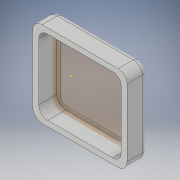
# Autodesk Inventor part: GoPro_Cap_Lens
Saved by Autodesk Inventor 2019 (Build 230136000, 136)
## iProperties
Created: 2019-02-06
Part Number: GoPro_Cap_Lens
Material: Generic
Document SubType Name: Modeling
Designer: jmc
Density: 1 g/cm^3
Appearance: Default
Author: jmc
## iProperties of the stored document GoPro_Cap_Lens_3DPrint.ipt
Created: 2019-02-06
Part Number: GoPro_Cap_Lens_3DPrint
Material: Generic
Document SubType Name: Modeling
Designer: assman
Density: 1 g/cm^3
Appearance: Default
Author: assman
Autodesk Inventor part; units mm, degrees
ref_plane "YZ Plane" through (0, 0, 0) normal (1, 0, 0) x (0, 1, 0)
ref_plane "XZ Plane" through (0, 0, 0) normal (0, 1, 0) x (-1, 0, 0)
ref_plane "XY Plane" through (0, 0, 0) normal (0, 0, 1) x (1, 0, 0)
sketch "Sketch1" plane through (-3.508, -14.003, 0) normal (0, 0, 1) x (1, 0, 0)
  line L0 (-3.495, 25.79953) -> (-3.495, 3.514145)
  line L1 (28.510999, 26.087) -> (28.510999, 3.154266)
  line L2 (0.019145, 0) -> (25.356733, 0)
  line L3 (25.487768, 29.005968) -> (-0.274, 29.005968)
  arc A0 (-3.495, 3.514145) -> (0.019145, 0) centre (0.019145, 3.514145) ccw
  arc A1 (25.356733, 0) -> (28.510999, 3.154266) centre (25.356733, 3.154266) ccw
  arc A2 (28.510999, 25.98277) -> (25.487768, 29.005968) centre (25.487768, 25.982737) ccw
  arc A3 (-0.274, 29.005968) -> (-3.495, 25.79953) centre (-0.288529, 25.79953) ccw
  line L4 (9.854411, 29.005968) -> (9.854411, 34.005968) construction
  point P0 (12.606884, 14.620633)
  dimension "d0" = 5
  constraints: 10 end point, 8 point on circle, 4 centre point, 2 point on line, 2 tangent, 1 vertical
  measures "d0" distance of L4.start L4.end
sketch "Sketch3" plane through (0, 0, 0) normal (0, 0, 1) x (1, 0, 0)
  arc A0 (-5.67549, 17.117612) -> (-9.369977, 13.439828) centre (-5.692155, 13.439828) ccw
  line L0 (-9.369977, 13.439828) -> (-9.369977, -12.121509)
  arc A1 (-9.369977, -12.121509) -> (-5.339252, -16.152233) centre (-5.339252, -12.121509) ccw
  line L1 (-5.339252, -16.152233) -> (23.722961, -16.152233)
  arc A2 (23.722961, -16.152233) -> (27.340904, -12.53429) centre (23.722961, -12.53429) ccw
  line L2 (27.340904, 13.769556) -> (27.340904, -12.53429)
  arc A3 (27.340904, 13.650004) -> (23.873258, 17.117612) centre (23.873258, 13.649966) ccw
  line L3 (23.873258, 17.117612) -> (-5.67549, 17.117612)
  point P0 (0, 0)
  point P1 (25.002999, 11.97977)
  point P2 (9.098884, 0.617633)
  constraints: 8 end point, 8 point on circle, 4 centre point, 1 point on line
extrude "Extrusion1" add sketch "Sketch3" along normal blind 7.886
shell "Shell1" thickness 2.5 removed faces 1 at (4.286172, 6.027663, 7.886)
ref_plane "Work Plane3" through (-5.682724, 14.617612, 2.5) normal (0, 0, 1) x (1, 0, 0)
sketch "Sketch4" plane through (-5.682724, 14.617612, 2.5) normal (0, 0, 1) x (1, 0, 0)
  point P0 (5.682724, -14.617612)
extrude "Extrusion2" cut sketch "Sketch1" along normal blind 21
sketch "Sketch5" plane through (-5.682724, 14.617612, 2.5) normal (0, 0, 1) x (1, 0, 0)
  arc A0 (0.362072, 0) -> (-1.187253, -1.907094) centre (1.886195, -2.821082) ccw
  line L0 (0.362072, 0) -> (0, 0)
  arc A1 (0, 0) -> (-1.187253, -1.177784) centre (-0.009431, -1.177784) ccw
  line L1 (-1.187253, -1.177784) -> (-1.187253, -1.907094)
  arc A2 (-1.187253, -26.064188) -> (0.663427, -28.269845) centre (2.19387, -25.106467) ccw
  line L2 (-1.187253, -26.064188) -> (-1.187253, -26.73912)
  arc A3 (-1.187253, -26.73912) -> (0.343472, -28.269845) centre (0.343472, -26.73912) ccw
  line L3 (0.343472, -28.269845) -> (0.663427, -28.269845)
  arc A4 (28.977067, -28.269845) -> (30.523628, -26.464498) centre (27.531457, -25.466346) ccw
  line L4 (28.977067, -28.269845) -> (29.405685, -28.269845)
  arc A5 (29.405685, -28.269845) -> (30.523628, -27.151902) centre (29.405685, -27.151902) ccw
  line L5 (30.523628, -27.151902) -> (30.523628, -26.464498)
  arc A6 (30.523628, -1.661234) -> (29.139496, 0) centre (27.662493, -2.637875) ccw
  line L6 (30.523628, -1.661234) -> (30.523628, -0.967608)
  arc A7 (30.523628, -0.967608) -> (29.555982, 0) centre (29.555983, -0.967646) ccw
  line L7 (29.555982, 0) -> (29.139496, 0)
  point P0 (5.682724, -14.617612)
extrude "Extrusion3" add sketch "Sketch5" along normal up to surface (5.386 mm away)
sketch "Sketch6" plane through (-5.682724, 14.617612, 2.5) normal (0, 0, 1) x (1, 0, 0)
  arc A0 (27.531457, -28.620612) -> (30.685723, -25.466346) centre (27.531457, -25.466346) ccw
  line L0 (2.19387, -28.620612) -> (27.531457, -28.620612)
  arc A1 (-1.320276, -25.106467) -> (2.19387, -28.620612) centre (2.19387, -25.106467) ccw
  line L1 (-1.320276, -2.821082) -> (-1.320276, -25.106467)
  arc A2 (1.900724, 0.385356) -> (-1.320276, -2.821082) centre (1.886195, -2.821082) ccw
  line L2 (27.662492, 0.385356) -> (1.900724, 0.385356)
  arc A3 (30.685723, -2.637842) -> (27.662492, 0.385356) centre (27.662493, -2.637875) ccw
  line L3 (30.685723, -25.466346) -> (30.685723, -2.637842)
  point P0 (5.682724, -14.617612)
extrude "Extrusion4" add sketch "Sketch6" against normal up to surface (2.5 mm away)
sketch "Sketch7" plane through (-5.682724, 14.617612, 2.5) normal (0, 0, 1) x (1, 0, 0)
  arc A0 (27.531457, -28.620612) -> (30.685723, -25.466346) centre (27.531457, -25.466346) ccw
  line L0 (30.685723, -2.637842) -> (30.685723, -25.466346)
  arc A1 (30.685723, -2.637842) -> (27.662492, 0.385356) centre (27.662493, -2.637875) ccw
  line L1 (1.900724, 0.385356) -> (27.662492, 0.385356)
  arc A2 (1.900724, 0.385356) -> (-1.320276, -2.821082) centre (1.886195, -2.821082) ccw
  line L2 (-1.320276, -25.106467) -> (-1.320276, -2.821082)
  arc A3 (-1.320276, -25.106467) -> (2.19387, -28.620612) centre (2.19387, -25.106467) ccw
  line L3 (27.531457, -28.620612) -> (2.19387, -28.620612)
  arc A4 (1.896794, -1.114644) -> (0.179724, -2.821082) centre (1.886195, -2.821082) ccw
  line L4 (1.896794, -1.114644) -> (27.662493, -1.114644)
  arc A5 (29.185723, -2.637875) -> (27.662493, -1.114644) centre (27.662493, -2.637875) ccw
  line L5 (29.185723, -2.637875) -> (29.185723, -25.466346)
  arc A6 (27.531457, -27.120612) -> (29.185723, -25.466346) centre (27.531457, -25.466346) ccw
  line L6 (27.531457, -27.120612) -> (2.19387, -27.120612)
  arc A7 (0.179724, -25.106467) -> (2.19387, -27.120612) centre (2.19387, -25.106467) ccw
  line L7 (0.179724, -25.106467) -> (0.179724, -2.821082)
  point P0 (5.682724, -14.617612)
  dimension "d11" = 1.5
  constraints: 8 end point, 8 point on circle, 4 centre point, 7 other
  measures "d11" radial gap between concentric circles of A2 A4
extrude "Extrusion5" cut sketch "Sketch7" against normal blind 21 contours L4 A5 L5 A6 L6 A7 L7 A4
sketch "Sketch8" plane through (-5.682724, 14.617612, 2.5) normal (0, 0, 1) x (1, 0, 0)
  line L0 (0.179724, -25.106467) -> (0.179724, -2.821082)
  arc A0 (1.896794, -1.114644) -> (0.179724, -2.821082) centre (1.886195, -2.821082) ccw
  line L1 (1.896794, -1.114644) -> (27.662493, -1.114644)
  arc A1 (29.185723, -2.637875) -> (27.662493, -1.114644) centre (27.662493, -2.637875) ccw
  line L2 (29.185723, -2.637875) -> (29.185723, -25.466346)
  arc A2 (27.531457, -27.120612) -> (29.185723, -25.466346) centre (27.531457, -25.466346) ccw
  line L3 (27.531457, -27.120612) -> (2.19387, -27.120612)
  arc A3 (0.179724, -25.106467) -> (2.19387, -27.120612) centre (2.19387, -25.106467) ccw
  arc A4 (27.531457, -28.620612) -> (30.685723, -25.466346) centre (27.531457, -25.466346) ccw
  line L4 (30.685723, -2.637842) -> (30.685723, -25.466346)
  arc A5 (30.685723, -2.637842) -> (27.662492, 0.385356) centre (27.662493, -2.637875) ccw
  line L5 (1.900724, 0.385356) -> (27.662492, 0.385356)
  arc A6 (1.900724, 0.385356) -> (-1.320276, -2.821082) centre (1.886195, -2.821082) ccw
  line L6 (-1.320276, -25.106467) -> (-1.320276, -2.821082)
  arc A7 (-1.320276, -25.106467) -> (2.19387, -28.620612) centre (2.19387, -25.106467) ccw
  line L7 (27.531457, -28.620612) -> (2.19387, -28.620612)
  point P0 (5.682724, -14.617612)
extrude "Extrusion6" cut sketch "Sketch8" against normal blind 1.6
fillet "Fillet1" radius 2 8 edges at (26.3252, 16.102, 0) (27.3409, 0.5579, 0) (26.2812, -15.0926, 0) (9.1919, -16.1522, 0) (-8.1894, -14.9717, 0) (-9.37, 0.6592, 0) (-8.2869, 16.0463, 0) (9.0989, 17.1176, 0)
fillet "Fillet1" radius 1 8 edges at (9.0969, 13.503, 0) (23.503, 0.5655, 0) (23.0185, -12.0185, 0) (9.1799, -12.503, 0) (-4.9131, -11.9131, 0) (-5.503, 0.6538, 0) (-4.9994, 13.0069, 0) (23.0569, 13.0568, 0)
body "Solid1"
